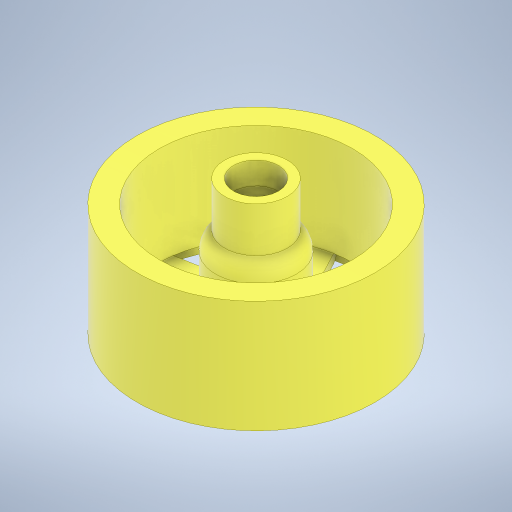
# Autodesk Inventor part: innertyre
Saved by Autodesk Inventor 2023 (Build 270158000, 158)
## iProperties
Created: 2022-11-29
Part Number: innertyre
Material: Generic
Document SubType Name: Modeling
Designer: kakik
Density: 1 g/cm^3
Appearance: Smooth - Yellow
Author: kakik
Autodesk Inventor part; units mm, degrees
ref_plane "YZ Plane" through (0, 0, 0) normal (1, 0, 0) x (0, 1, 0)
ref_plane "XZ Plane" through (0, 0, 0) normal (0, 1, 0) x (-1, 0, 0)
ref_plane "XY Plane" through (0, 0, 0) normal (0, 0, 1) x (1, 0, 0)
sketch "Sketch1" plane through (0, 0, 0) normal (0, 1, 0) x (-1, 0, 0)
  circle A0 centre (0, 0) radius 26.5
  dimension "d0" = 53
  constraints: 1 centre point, 1 coincident
  measures "d0" diameter of A0
extrude "Extrusion1" add sketch "Sketch1" along normal blind 25
sketch "Sketch2" plane through (0, 0, 0) normal (0, -1, 0) x (1, 0, 0)
  circle A0 centre (0, 0) radius 26.5 projected
  circle A1 centre (0, 0) radius 23.5
  dimension "d3" = 3
  constraints: 1 centre point
  measures "d3" radial gap between concentric circles of A0 A1
extrude "Extrusion2" cut sketch "Sketch2" against normal blind 3 contours A1
sketch "Sketch4" plane through (0, 3, 0) normal (0, -1, 0) x (1, 0, 0)
  circle A0 centre (0, 0) radius 23.5 projected
  circle A1 centre (0, 0) radius 21.5
  dimension "d13" = 2
  constraints: 1 centre point
  measures "d13" radial gap between concentric circles of A0 A1
sketch "Sketch3" plane through (0, 3, 0) normal (0, -1, 0) x (1, 0, 0)
  circle A0 centre (0, 0) radius 23.5 projected
  line L0 (0, 0) -> (-26.5, 0) construction
  circle A1 centre (0, 0) radius 26.5 projected
  line L1 (0, 0) -> (0, 6.6202)
  line L2 (0, 6.6202) -> (-23.3666, 2.5)
  line L3 (0, 0) -> (0, -6.6202)
  line L4 (0, -6.6202) -> (-23.3666, -2.5)
  dimension "d11" = 5
  dimension "d12" = 80
  constraints: 10 end point, 2 point on circle, 1 collinear, 1 horizontal, 1 horizontal alignment, 1 point on line, 1 vertical, 2 other
  measures "d11" distance of L2.end L4.end
  measures "d12" angle of L3 L4
extrude "Extrusion3" add sketch "Sketch3" along normal blind 2 contours L2 L1 L3 L4 A0 picked at (-7.7889, -3.0401)
pattern_circular "Circular Pattern1" count 5 over 360 about axis through (0, 0, 0) along (0, 1, 0) of "Extrusion3"
extrude "Extrusion4" cut sketch "Sketch4" against normal through all contours A1
sketch "Sketch6" plane through (0, 0, 0) normal (0, 0, 1) x (1, 0, 0)
  line L0 (-23.5, 0) -> (-23.5, 1) projected
  line L1 (-9.5983, 3) -> (-23.3666, 3) projected
  line L2 (-23.3666, 1) -> (-23.5, 1) projected
  line L3 (-23.5, 3) -> (-23.5, 3)
  line L4 (-23.5, 3) -> (-14.0664, 3)
  line L5 (-7.3324, 1) -> (-23.3666, 1) projected
  line L6 (-14.0664, 1) -> (-21.5, 1)
  arc A0 (-23.5, 3) -> (-21.5, 1) centre (-21.5, 3) ccw
  line L7 (-23.5, 1) -> (-23.5, 3)
  line L8 (-23.5, 1) -> (-21.5, 1)
  line L9 (0, -5) -> (0, 30) projected
  point P0 (0, 0)
  dimension "d16" = 2
  constraints: 10 end point, 4 point on line, 4 tangent, 2 point on circle, 2 vertical, 1 centre point, 1 collinear, 1 perpendicular
  measures "d16" radius of A0
revolve "Revolution1" cut sketch "Sketch6" angle 360 about axis through (0, -10, 0) along (0, 1, 0)
fillet "Fillet1" radius 7 1 edges at (-7.3324, 2, -5.3273)
pattern_circular "Circular Pattern2" count 5 over 360 about axis through (0, 0, 0) along (0, 1, 0) of "Fillet1"
sketch "Sketch8" plane through (0, 3, 0) normal (0, 1, 0) x (1, 0, 0)
  circle A0 centre (0, 0) radius 9
  dimension "d27" = 18
  constraints: 1 centre point, 1 coincident
  measures "d27" diameter of A0
sketch "Sketch7" plane through (0, 1, 0) normal (0, -1, 0) x (1, 0, 0)
  circle A0 centre (0, 0) radius 6.5
  circle A1 centre (0, 0) radius 5
  circle A2 centre (0, 0) radius 9
  dimension "d22" = 13
  dimension "d23" = 1.5
  dimension "d26" = 18
  constraints: 3 centre point, 2 coincident
  measures "d22" diameter of A0
  measures "d23" radial gap between concentric circles of A0 A1
  measures "d26" diameter of A2
extrude "Extrusion5" cut sketch "Sketch7" against normal blind 5 contours A0 | A1
extrude "Extrusion6" add sketch "Sketch8" along normal up to surface (22 mm away)
sketch "Sketch9" plane through (0, 0, 0) normal (1, 0, 0) x (0, 1, 0)
  line L0 (1, 6.5) -> (3, 6.5) projected
  line L1 (3, 6.5) -> (3, 5)
  line L2 (3, 4.8626) -> (1, 4.8626) projected
  line L3 (3, 5) -> (1, 6.5)
  line L4 (1, 4.8626) -> (1, 10.2087) projected
  line L5 (3, 6.5) -> (1, 6.5)
  line L6 (3, -10.2087) -> (3, 10.2087) projected
  line L7 (-5, 0) -> (30, 0) projected
  point P0 (0, 0)
  dimension "d30" = 1.5
  constraints: 6 end point, 2 perpendicular, 2 point on line
  measures "d30" distance of L1.start L1.end
revolve "Revolution2" add sketch "Sketch9" angle 360 about axis through (0, -10, 0) along (0, 1, 0) contours L0 L1 L3
sketch "Sketch10" plane through (0, 3, 0) normal (0, -1, 0) x (1, 0, 0)
  circle A0 centre (0, 0) radius 3.5
  dimension "d32" = 7
  constraints: 1 centre point, 1 coincident
  measures "d32" diameter of A0
extrude "Extrusion7" add sketch "Sketch10" along normal blind 1
sketch "Sketch11" plane through (0, 3, 0) normal (0, -1, 0) x (1, 0, 0)
  circle A0 centre (0, 0) radius 3.5 projected
  line L0 (-3.5, 0) -> (-5, 0)
  circle A1 centre (0, 0) radius 5 projected
  circle A2 centre (-4.25, 0) radius 0.3333
  constraints: 2 end point, 2 horizontal alignment, 1 centre point, 1 horizontal, 1 midpoint, 2 other
extrude "Extrusion8" add sketch "Sketch11" along normal blind 1 contours A2 L0 | L0 A2
pattern_circular "Circular Pattern3" count 4 over 360 about axis through (0, 2, 0) along (0, -1, 0) of "Extrusion8"
sketch "Sketch12" plane through (0, 1, 0) normal (0, -1, 0) x (1, 0, 0)
  arc A0 (-15, -1) -> (-15, 1) centre (-15, 0) ccw
  line L0 (-15, 1) -> (-15, -1)
  circle A1 centre (0, 0) radius 23.5 projected
  dimension "d40" = 2
  dimension "d42" = 15
  constraints: 2 end point, 2 point on circle, 1 centre point, 1 midpoint, 1 vertical
  measures "d40" diameter of A0
  measures "d42" distance of A1.centre point (-15, 0)
revolve "Revolution3" cut sketch "Sketch12" angle 360 about axis through (-15, 1, 1) along (0, 0, -1) contours L0 A0
pattern_circular "Circular Pattern4" count 5 over 360 about axis through (0, 0, 0) along (0, 1, 0) of "Revolution3"
sketch "Sketch13" plane through (0, 25, 0) normal (0, 1, 0) x (1, 0, 0)
  circle A0 centre (0, 0) radius 5
  circle A1 centre (0, 0) radius 7
  dimension "d46" = 10
  dimension "d47" = 2
  constraints: 2 centre point, 1 coincident
  measures "d46" diameter of A0
  measures "d47" radial gap between concentric circles of A0 A1
extrude "Extrusion9" add sketch "Sketch13" along normal blind 5
sketch "Sketch14" plane through (0, 25, 0) normal (0, 1, 0) x (1, 0, 0)
  circle A0 centre (0, 0) radius 9 projected
  circle A1 centre (0, 0) radius 7 projected
extrude "Extrusion10" cut sketch "Sketch14" against normal blind 5
fillet "Fillet2" radius 5 1 edges at (-9, 20, 0)
body "Solid1"
